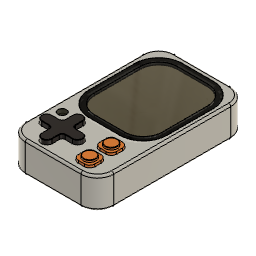
MVP Mecanico v1 (Autodesk Fusion 360 design; units mm, degrees)
Autodesk Fusion 360 part; units mm, degrees
(part 1 of 2)
sketch "Boceto1" plane through (0, 0, 0) normal (0, 0, 1) x (1, 0, 0)
  line L0 (7.34, -20.255) -> (-7.34, -20.255)
  line L1 (-16.54, -11.055) -> (-16.54, 11.055)
  line L2 (-7.34, 20.255) -> (7.34, 20.255)
  line L3 (16.54, 11.055) -> (16.54, -11.055)
  line L4 (16.54, -20.255) -> (-16.54, 20.255) construction
  line L5 (-16.54, -20.255) -> (16.54, 20.255) construction
  line L6 (8.265, -22.225) -> (-8.265, -22.225)
  line L7 (-17.465, -13.025) -> (-17.465, 11.855)
  line L8 (-8.265, 21.055) -> (8.265, 21.055)
  line L9 (17.465, 11.855) -> (17.465, -13.025)
  arc A0 (-7.34, 20.255) -> (-16.54, 11.055) centre (-7.34, 11.055) ccw
  arc A1 (16.54, 11.055) -> (7.34, 20.255) centre (7.34, 11.055) ccw
  arc A2 (-16.54, -11.055) -> (-7.34, -20.255) centre (-7.34, -11.055) ccw
  arc A3 (7.34, -20.255) -> (16.54, -11.055) centre (7.34, -11.055) ccw
  arc A4 (-8.265, 21.055) -> (-17.465, 11.855) centre (-8.265, 11.855) ccw
  arc A5 (17.465, 11.855) -> (8.265, 21.055) centre (8.265, 11.855) ccw
  arc A6 (-17.465, -13.025) -> (-8.265, -22.225) centre (-8.265, -13.025) ccw
  arc A7 (8.265, -22.225) -> (17.465, -13.025) centre (8.265, -13.025) ccw
  dimension "d3" = 33.08
  dimension "d4" = 40.51
  dimension "d7" = 9.2
  dimension "d8" = 9.2
  dimension "d9" = 9.2
  dimension "d10" = 9.2
  dimension "d11" = 9.2
  dimension "d12" = 9.2
  dimension "d13" = 9.2
  dimension "d14" = 9.2
  dimension "d15" = 0.8
  dimension "d16" = 43.28
  dimension "d17" = 34.93
  dimension "d18" = 0.925
  constraint horizontal L0
  constraint perpendicular L0 L1
  constraint parallel L0 L2
  constraint parallel L1 L3
  constraint coincident L4 origin
  constraint coincident L5 origin
  constraint horizontal L6
  constraint perpendicular L6 L7
  constraint parallel L6 L8
  constraint parallel L7 L9
  constraint coincident L4.end L1
  constraint coincident L4.end L2
  constraint tangent L1 A0
  constraint tangent L2 A0
  constraint coincident L5.end L2
  constraint coincident L5.end L3
  constraint tangent L2 A1
  constraint tangent L3 A1
  constraint coincident L5.start L1
  constraint coincident L5.start L0
  constraint tangent L1 A2
  constraint tangent L0 A2
  constraint coincident L4.start L0
  constraint coincident L4.start L3
  constraint tangent L0 A3
  constraint tangent L3 A3
  constraint tangent L7 A4
  constraint tangent L8 A4
  constraint tangent L8 A5
  constraint tangent L9 A5
  constraint tangent L7 A6
  constraint tangent L6 A6
  constraint tangent L6 A7
  constraint tangent L9 A7
  measures "d3" distance of L4.end L5.end
  measures "d4" distance of L5.start L4.end
  measures "d7" radius of A0
  measures "d8" radius of A1
  measures "d9" radius of A2
  measures "d10" radius of A3
  measures "d11" radius of A4
  measures "d12" radius of A5
  measures "d13" radius of A6
  measures "d14" radius of A7
  measures "d15" distance of L2 L8
  measures "d16" distance of L6 L8
  measures "d17" distance of L7 L9
  measures "d18" distance of L1 L7
extrude "Extruir1" add sketch "Boceto1" along normal blind 0.83 makes body 1
extrude "Extruir2" add sketch "Boceto1" along normal blind 1.03 contours L0 L1 L2 L3 A0 A1 A2 A3 bodies 1
sketch "Boceto2" plane through (0, 0, 1.03) normal (0, 0, 1) x (-1, 0, 0)
  line L0 (-7.395, 20.305) -> (7.395, 20.305)
  line L1 (16.595, 11.105) -> (16.595, -11.105)
  line L2 (7.395, -20.305) -> (-7.395, -20.305)
  line L3 (-16.595, -11.105) -> (-16.595, 11.105)
  line L4 (-16.595, 20.305) -> (16.595, -20.305) construction
  line L5 (16.595, 20.305) -> (-16.595, -20.305) construction
  arc A0 (7.395, -20.305) -> (16.595, -11.105) centre (7.395, -11.105) ccw
  arc A1 (-16.595, -11.105) -> (-7.395, -20.305) centre (-7.395, -11.105) ccw
  arc A2 (16.595, 11.105) -> (7.395, 20.305) centre (7.395, 11.105) ccw
  arc A3 (-7.395, 20.305) -> (-16.595, 11.105) centre (-7.395, 11.105) ccw
  line L6 (-7.545, 22.755) -> (7.545, 22.755)
  line L7 (19.045, 11.255) -> (19.045, -11.255)
  line L8 (7.545, -22.755) -> (-7.545, -22.755)
  line L9 (-19.045, -11.255) -> (-19.045, 11.255)
  line L10 (-19.045, 22.755) -> (19.045, -22.755) construction
  line L11 (19.045, 22.755) -> (-19.045, -22.755) construction
  arc A4 (7.545, -22.755) -> (19.045, -11.255) centre (7.545, -11.255) ccw
  arc A5 (-19.045, -11.255) -> (-7.545, -22.755) centre (-7.545, -11.255) ccw
  arc A6 (19.045, 11.255) -> (7.545, 22.755) centre (7.545, 11.255) ccw
  arc A7 (-7.545, 22.755) -> (-19.045, 11.255) centre (-7.545, 11.255) ccw
  dimension "d30" = 40.61
  dimension "d31" = 33.19
  dimension "d32" = 9.2
  dimension "d33" = 9.2
  dimension "d34" = 9.2
  dimension "d35" = 9.2
  dimension "d36" = 45.51
  dimension "d37" = 38.09
  dimension "d38" = 11.5
  dimension "d39" = 11.5
  dimension "d40" = 11.5
  dimension "d41" = 11.5
  constraint horizontal L0
  constraint perpendicular L0 L1
  constraint parallel L0 L2
  constraint parallel L1 L3
  constraint coincident L4 origin
  constraint coincident L5 origin
  constraint coincident L4.end L1
  constraint coincident L4.end L2
  constraint tangent L1 A0
  constraint tangent L2 A0
  constraint coincident L5.end L2
  constraint coincident L5.end L3
  constraint tangent L2 A1
  constraint tangent L3 A1
  constraint coincident L5.start L1
  constraint coincident L5.start L0
  constraint tangent L1 A2
  constraint tangent L0 A2
  constraint coincident L4.start L0
  constraint coincident L4.start L3
  constraint tangent L0 A3
  constraint tangent L3 A3
  constraint horizontal L6
  constraint perpendicular L6 L7
  constraint parallel L6 L8
  constraint parallel L7 L9
  constraint coincident L10 origin
  constraint coincident L11 origin
  constraint coincident L10.end L7
  constraint coincident L10.end L8
  constraint tangent L7 A4
  constraint tangent L8 A4
  constraint coincident L11.end L8
  constraint coincident L11.end L9
  constraint tangent L8 A5
  constraint tangent L9 A5
  constraint coincident L11.start L7
  constraint coincident L11.start L6
  constraint tangent L7 A6
  constraint tangent L6 A6
  constraint coincident L10.start L6
  constraint coincident L10.start L9
  constraint tangent L6 A7
  constraint tangent L9 A7
  measures "d30" distance of L5.start L4.end
  measures "d31" distance of L4.end L5.end
  measures "d32" radius of A0
  measures "d33" radius of A1
  measures "d34" radius of A2
  measures "d35" radius of A3
  measures "d36" distance of L11.start L10.end
  measures "d37" distance of L10.end L11.end
  measures "d38" radius of A4
  measures "d39" radius of A5
  measures "d40" radius of A6
  measures "d41" radius of A7
sketch "Boceto3" plane through (0, 0, 0.83) normal (0, 0, 1) x (-1, 0, 0)
  arc A0 (17.465, 13.025) -> (8.265, 22.225) centre (8.265, 13.025) ccw
  line L0 (8.265, 22.225) -> (-8.265, 22.225)
  arc A1 (-8.265, 22.225) -> (-17.465, 13.025) centre (-8.265, 13.025) ccw
  line L1 (-17.465, 13.025) -> (-17.465, -11.855)
  arc A2 (-17.465, -11.855) -> (-8.265, -21.055) centre (-8.265, -11.855) ccw
  line L2 (-8.265, -21.055) -> (8.265, -21.055)
  arc A3 (8.265, -21.055) -> (17.465, -11.855) centre (8.265, -11.855) ccw
  line L3 (17.465, -11.855) -> (17.465, 13.025)
  line L4 (11.3983, 21.675) -> (-11.3983, 21.675)
  arc A4 (16.54, 11.055) -> (7.34, 20.255) centre (7.34, 11.055) ccw
  line L5 (16.54, 11.055) -> (16.54, -11.055)
  arc A5 (7.34, -20.255) -> (16.54, -11.055) centre (7.34, -11.055) ccw
  line L6 (7.34, -20.255) -> (-7.34, -20.255)
  arc A6 (-16.54, -11.055) -> (-7.34, -20.255) centre (-7.34, -11.055) ccw
  line L7 (-16.54, -11.055) -> (-16.54, 11.055)
  arc A7 (-7.34, 20.255) -> (-16.54, 11.055) centre (-7.34, 11.055) ccw
  line L8 (-7.34, 20.255) -> (7.34, 20.255)
  dimension "d42" = 0.55
  constraint coincident A0 L4.start
  constraint coincident A1 L4.end
  constraint horizontal L4
  measures "d42" distance of L0 L4
extrude "Extruir3" cut sketch "Boceto3" against normal blind 0.4 contours A0 L0 A1 L4 bodies 1
extrude "Extruir4" add sketch "Boceto2" along normal blind 1.1 separate body makes body 2
extrude "Extruir5" add 1 faces at (-5.5133, -3.685, 1.03) along direction (0, 0, 1) blind 1.1 separate body on bodies 1 makes body 3
sketch "Boceto4" plane through (0, 0, 1.03) normal (0, 0, -1) x (1, 0, 0)
  arc A0 (-7.395, 20.305) -> (-16.595, 11.105) centre (-7.395, 11.105) ccw
  line L0 (-7.395, 20.305) -> (7.395, 20.305)
  arc A1 (16.595, 11.105) -> (7.395, 20.305) centre (7.395, 11.105) ccw
  line L1 (16.595, 11.105) -> (16.595, -11.105)
  arc A2 (7.395, -20.305) -> (16.595, -11.105) centre (7.395, -11.105) ccw
  line L2 (7.395, -20.305) -> (-7.395, -20.305)
  arc A3 (-16.595, -11.105) -> (-7.395, -20.305) centre (-7.395, -11.105) ccw
  line L3 (-16.595, -11.105) -> (-16.595, 11.105)
  arc A4 (-7.545, 22.755) -> (-19.045, 11.255) centre (-7.545, 11.255) ccw
  line L4 (-19.045, 11.255) -> (-19.045, -11.255)
  arc A5 (-19.045, -11.255) -> (-7.545, -22.755) centre (-7.545, -11.255) ccw
  line L5 (-7.545, -22.755) -> (7.545, -22.755)
  arc A6 (7.545, -22.755) -> (19.045, -11.255) centre (7.545, -11.255) ccw
  line L6 (19.045, -11.255) -> (19.045, 11.255)
  arc A7 (19.045, 11.255) -> (7.545, 22.755) centre (7.545, 11.255) ccw
  line L7 (7.545, 22.755) -> (-7.545, 22.755)
  line L8 (-8.265, 22.425) -> (8.265, 22.425)
  line L9 (17.665, 13.025) -> (17.665, -11.855)
  line L10 (8.265, -21.255) -> (-8.265, -21.255)
  line L11 (-17.665, -11.855) -> (-17.665, 13.025)
  line L12 (8.265, 22.225) -> (-8.265, 22.225)
  arc A8 (8.265, -21.255) -> (17.665, -11.855) centre (8.265, -11.855) ccw
  arc A9 (-17.665, -11.855) -> (-8.265, -21.255) centre (-8.265, -11.855) ccw
  arc A10 (17.665, 13.025) -> (8.265, 22.425) centre (8.265, 13.025) ccw
  arc A11 (-8.265, 22.425) -> (-17.665, 13.025) centre (-8.265, 13.025) ccw
  line L13 (-8.45, 25) -> (8.45, 25)
  line L14 (20, 13.45) -> (20, -13.45)
  line L15 (8.45, -25) -> (-8.45, -25)
  line L16 (-20, -13.45) -> (-20, 13.45)
  line L17 (-20, 25) -> (20, -25) construction
  line L18 (20, 25) -> (-20, -25) construction
  arc A12 (20, 13.45) -> (8.45, 25) centre (8.45, 13.45) ccw
  arc A13 (-8.45, 25) -> (-20, 13.45) centre (-8.45, 13.45) ccw
  arc A14 (8.45, -25) -> (20, -13.45) centre (8.45, -13.45) ccw
  arc A15 (-20, -13.45) -> (-8.45, -25) centre (-8.45, -13.45) ccw
  dimension "d52" = 0.2
  dimension "d55" = 9.4
  dimension "d56" = 9.4
  dimension "d57" = 9.4
  dimension "d58" = 9.4
  dimension "d59" = 40
  dimension "d60" = 50
  dimension "d61" = 11.55
  dimension "d62" = 11.55
  dimension "d63" = 11.55
  dimension "d64" = 11.55
  constraint horizontal L8
  constraint perpendicular L8 L9
  constraint parallel L8 L10
  constraint parallel L9 L11
  constraint tangent L9 A8
  constraint tangent L10 A8
  constraint tangent L10 A9
  constraint tangent L11 A9
  constraint tangent L9 A10
  constraint tangent L8 A10
  constraint tangent L8 A11
  constraint tangent L11 A11
  constraint horizontal L13
  constraint perpendicular L13 L14
  constraint parallel L13 L15
  constraint parallel L14 L16
  constraint coincident L17 origin
  constraint coincident L18 origin
  constraint coincident L18.start L14
  constraint coincident L18.start L13
  constraint tangent L14 A12
  constraint tangent L13 A12
  constraint coincident L17.start L13
  constraint coincident L17.start L16
  constraint tangent L13 A13
  constraint tangent L16 A13
  constraint coincident L17.end L15
  constraint coincident L17.end L14
  constraint tangent L15 A14
  constraint tangent L14 A14
  constraint coincident L18.end L15
  constraint coincident L18.end L16
  constraint tangent L15 A15
  constraint tangent L16 A15
  measures "d52" distance of L8 L12
  measures "d55" radius of A8
  measures "d56" radius of A9
  measures "d57" radius of A10
  measures "d58" radius of A11
  measures "d59" distance of L17.end L18.end
  measures "d60" distance of L18.start L17.end
  measures "d61" radius of A12
  measures "d62" radius of A13
  measures "d63" radius of A14
  measures "d64" radius of A15
sketch "Boceto5" plane through (0, 0, 2.13) normal (0, 0, 1) x (-1, 0, 0)
  arc A0 (16.595, 11.105) -> (7.395, 20.305) centre (7.395, 11.105) ccw
  line L0 (16.595, 11.105) -> (16.595, -11.105)
  arc A1 (7.395, -20.305) -> (16.595, -11.105) centre (7.395, -11.105) ccw
  line L1 (7.395, -20.305) -> (-7.395, -20.305)
  arc A2 (-16.595, -11.105) -> (-7.395, -20.305) centre (-7.395, -11.105) ccw
  line L2 (-16.595, -11.105) -> (-16.595, 11.105)
  arc A3 (-7.395, 20.305) -> (-16.595, 11.105) centre (-7.395, 11.105) ccw
  line L3 (-7.395, 20.305) -> (7.395, 20.305)
  arc A4 (19.045, 11.255) -> (7.545, 22.755) centre (7.545, 11.255) ccw
  line L4 (7.545, 22.755) -> (-7.545, 22.755)
  arc A5 (-7.545, 22.755) -> (-19.045, 11.255) centre (-7.545, 11.255) ccw
  line L5 (-19.045, 11.255) -> (-19.045, -11.255)
  arc A6 (-19.045, -11.255) -> (-7.545, -22.755) centre (-7.545, -11.255) ccw
  line L6 (-7.545, -22.755) -> (7.545, -22.755)
  arc A7 (7.545, -22.755) -> (19.045, -11.255) centre (7.545, -11.255) ccw
  line L7 (19.045, -11.255) -> (19.045, 11.255)
  line L8 (-7.57, 22.83) -> (7.57, 22.83)
  line L9 (19.12, 11.28) -> (19.12, -11.28)
  line L10 (7.57, -22.83) -> (-7.57, -22.83)
  line L11 (-19.12, -11.28) -> (-19.12, 11.28)
  line L12 (-19.12, 22.83) -> (19.12, -22.83) construction
  line L13 (19.12, 22.83) -> (-19.12, -22.83) construction
  arc A8 (7.57, -22.83) -> (19.12, -11.28) centre (7.57, -11.28) ccw
  arc A9 (-19.12, -11.28) -> (-7.57, -22.83) centre (-7.57, -11.28) ccw
  arc A10 (19.12, 11.28) -> (7.57, 22.83) centre (7.57, 11.28) ccw
  arc A11 (-7.57, 22.83) -> (-19.12, 11.28) centre (-7.57, 11.28) ccw
  line L14 (-13.52, -25.28) -> (13.57, -25.28)
  line L15 (21.57, -17.28) -> (21.57, 39.73)
  line L16 (13.57, 47.73) -> (-13.52, 47.73)
  line L17 (-21.52, 39.73) -> (-21.52, -17.28)
  line L18 (-21.52, -25.28) -> (21.57, 47.73) construction
  line L19 (21.57, -25.28) -> (-21.52, 47.73) construction
  arc A12 (13.57, -25.28) -> (21.57, -17.28) centre (13.57, -17.28) ccw
  arc A13 (-21.52, -17.28) -> (-13.52, -25.28) centre (-13.52, -17.28) ccw
  arc A14 (21.57, 39.73) -> (13.57, 47.73) centre (13.57, 39.73) ccw
  arc A15 (-13.52, 47.73) -> (-21.52, 39.73) centre (-13.52, 39.73) ccw
  point P0 (0.025, 11.225)
  dimension "d67" = 45.66
  dimension "d68" = 38.24
  dimension "d69" = 11.55
  dimension "d70" = 11.55
  dimension "d71" = 11.55
  dimension "d72" = 11.55
  dimension "d76" = 73.01
  dimension "d77" = 8
  dimension "d78" = 8
  dimension "d79" = 8
  dimension "d80" = 8
  dimension "d234" = 43.09
  constraint horizontal L8
  constraint perpendicular L8 L9
  constraint parallel L8 L10
  constraint parallel L9 L11
  constraint coincident L12 origin
  constraint coincident L13 origin
  constraint coincident L12.end L9
  constraint coincident L12.end L10
  constraint tangent L9 A8
  constraint tangent L10 A8
  constraint coincident L13.end L10
  constraint coincident L13.end L11
  constraint tangent L10 A9
  constraint tangent L11 A9
  constraint coincident L13.start L9
  constraint coincident L13.start L8
  constraint tangent L9 A10
  constraint tangent L8 A10
  constraint coincident L12.start L8
  constraint coincident L12.start L11
  constraint tangent L8 A11
  constraint tangent L11 A11
  constraint horizontal L14
  constraint perpendicular L14 L15
  constraint parallel L14 L16
  constraint parallel L15 L17
  constraint coincident L18 P0
  constraint coincident L19 P0
  constraint coincident L19.start L15
  constraint coincident L19.start L14
  constraint tangent L15 A12
  constraint tangent L14 A12
  constraint coincident L18.start L14
  constraint coincident L18.start L17
  constraint tangent L14 A13
  constraint tangent L17 A13
  constraint coincident L18.end L15
  constraint coincident L18.end L16
  constraint tangent L15 A14
  constraint tangent L16 A14
  constraint coincident L19.end L17
  constraint coincident L19.end L16
  constraint tangent L17 A15
  constraint tangent L16 A15
  measures "d67" distance of L13.start L12.end
  measures "d68" distance of L12.end L13.end
  measures "d69" radius of A8
  measures "d70" radius of A9
  measures "d71" radius of A10
  measures "d72" radius of A11
  measures "d76" distance of L19.start L18.end
  measures "d77" radius of A12
  measures "d78" radius of A13
  measures "d79" radius of A14
  measures "d80" radius of A15
  measures "d234" distance of L15 L17
extrude "Extruir7" add sketch "Boceto5" against normal blind 2 separate body contours L14 L15 L16 L17 A12 A13 A14 A15 makes body 4
sketch "Boceto6" plane through (0, 0, 0.13) normal (0, 0, -1) x (1, 0, 0)
  arc A0 (-7.57, 22.83) -> (-19.12, 11.28) centre (-7.57, 11.28) ccw
  line L0 (-7.57, 22.83) -> (7.57, 22.83)
  arc A1 (19.12, 11.28) -> (7.57, 22.83) centre (7.57, 11.28) ccw
  line L1 (19.12, 11.28) -> (19.12, -11.28)
  arc A2 (7.57, -22.83) -> (19.12, -11.28) centre (7.57, -11.28) ccw
  line L2 (7.57, -22.83) -> (-7.57, -22.83)
  arc A3 (-19.12, -11.28) -> (-7.57, -22.83) centre (-7.57, -11.28) ccw
  line L3 (-19.12, -11.28) -> (-19.12, 11.28)
  arc A4 (21.52, 39.73) -> (13.52, 47.73) centre (13.52, 39.73) ccw
  line L4 (13.52, 47.73) -> (-13.57, 47.73)
  arc A5 (-13.57, 47.73) -> (-21.57, 39.73) centre (-13.57, 39.73) ccw
  line L5 (-21.57, 39.73) -> (-21.57, -17.28)
  arc A6 (-21.57, -17.28) -> (-13.57, -25.28) centre (-13.57, -17.28) ccw
  line L6 (-13.57, -25.28) -> (13.52, -25.28)
  arc A7 (13.52, -25.28) -> (21.52, -17.28) centre (13.52, -17.28) ccw
  line L7 (21.52, -17.28) -> (21.52, 39.73)
  line L8 (-13.57, -23.78) -> (13.52, -23.78)
  arc A8 (13.52, -23.78) -> (20.02, -17.28) centre (13.52, -17.28) ccw
  line L9 (20.02, -17.28) -> (20.02, 39.73)
  arc A9 (20.02, 39.73) -> (13.52, 46.23) centre (13.52, 39.73) ccw
  line L10 (13.52, 46.23) -> (-13.57, 46.23)
  arc A10 (-13.57, 46.23) -> (-20.07, 39.73) centre (-13.57, 39.73) ccw
  line L11 (-20.07, 39.73) -> (-20.07, -17.28)
  arc A11 (-20.07, -17.28) -> (-13.57, -23.78) centre (-13.57, -17.28) ccw
  dimension "d83" = -1.5
extrude "Extruir8" add sketch "Boceto6" along normal blind 13 contours A4 L4 A5 L5 A6 L6 A7 L7 bodies 4
fillet "Empalme1" radius 1 8 edges at (21.52, -11.225, 2.13) (19.1769, 22.9369, 2.13) (-0.025, 25.28, 2.13) (-19.2269, 22.9369, 2.13) (-21.57, -11.225, 2.13) (-19.2269, -45.3869, 2.13) (-0.025, -47.73, 2.13) (19.1769, -45.3869, 2.13) on bodies 4
fillet "Empalme2" radius 1 8 edges at (-21.57, -11.225, -12.87) (-19.2269, 22.9369, -12.87) (-0.025, 25.28, -12.87) (19.1769, 22.9369, -12.87) (21.52, -11.225, -12.87) (19.1769, -45.3869, -12.87) (-0.025, -47.73, -12.87) (-19.2269, -45.3869, -12.87) on bodies 4
extrude "Extruir9" add sketch "Boceto4" along normal up to surface (0.9 mm away) separate body contours A4 L4 A5 L5 A6 L6 A7 L7 | L13 L14 L15 L16 A12 A13 A14 A15 makes body 5
ref_plane "PlanoDeObra1" through (-0.025, -11.225, -10.34) normal (0, 0, -1) x (1, 0, 0)
sketch "Boceto7" plane through (0, 0, -10.34) normal (0, 0, -1) x (-1, 0, 0)
  line L0 (-13.52, -47.73) -> (13.57, -47.73)
  line L1 (-21.52, 17.28) -> (-21.52, -39.73)
  circle A0 centre (-15.52, -41.73) radius 1.4
  line L2 (20.07, -11.225) -> (-20.02, -11.225) construction
  line L3 (-20.02, -39.73) -> (-20.02, 17.28)
  line L4 (20.07, 17.28) -> (20.07, -39.73)
  line L5 (0.025, -46.23) -> (0.025, 23.78) construction
  line L6 (13.57, -46.23) -> (-13.52, -46.23)
  line L7 (-13.52, 23.78) -> (13.57, 23.78)
  line L8 (-13.52, -46.23) -> (-20.02, -46.23) construction
  line L9 (-20.02, -39.73) -> (-20.02, -46.23) construction
  line L10 (-20.02, -46.23) -> (-16.036, -42.6017) construction
  line L11 (-13.5, -43.948) -> (-17.54, -39.512) construction
  arc A1 (-13.5, -43.948) -> (-17.54, -39.512) centre (-15.52, -41.73) ccw
  arc A2 (-20.02, -39.73) -> (-13.52, -46.23) centre (-14.0388, -40.2488) ccw
  line L12 (-13.5, -43.948) -> (-15.7552, -46.0019)
  line L13 (-17.54, -39.512) -> (-19.8786, -41.6418)
  circle A3 centre (-15.52, 19.28) radius 1.4
  line L14 (-13.5, 21.498) -> (-15.7552, 23.5519)
  arc A4 (-17.54, 17.062) -> (-13.5, 21.498) centre (-15.52, 19.28) ccw
  line L15 (-17.54, 17.062) -> (-19.8786, 19.1918)
  arc A5 (-13.52, 23.78) -> (-20.02, 17.28) centre (-14.0388, 17.7988) ccw
  circle A6 centre (15.57, 19.28) radius 1.4
  line L16 (17.59, 17.062) -> (19.9286, 19.1918)
  arc A7 (13.55, 21.498) -> (17.59, 17.062) centre (15.57, 19.28) ccw
  line L17 (13.55, 21.498) -> (15.8052, 23.5519)
  arc A8 (20.07, 17.28) -> (13.57, 23.78) centre (14.0888, 17.7988) ccw
  line L18 (13.55, -43.948) -> (15.8052, -46.0019)
  arc A9 (17.59, -39.512) -> (13.55, -43.948) centre (15.57, -41.73) ccw
  circle A10 centre (15.57, -41.73) radius 1.4
  line L19 (17.59, -39.512) -> (19.9286, -41.6418)
  arc A11 (13.57, -46.23) -> (20.07, -39.73) centre (14.0888, -40.2488) ccw
  dimension "d93" = 6
  dimension "d94" = 6
  dimension "d96" = 2.8
  dimension "d97" = 6
  constraint horizontal L2
  constraint midpoint L2.end L3
  constraint coincident L2.start L4
  constraint vertical L5
  constraint midpoint L5.start L6
  constraint midpoint L5.end L7
  constraint concentric A0 A1
  constraint coincident L6.end L8.start
  constraint parallel L6 L8
  constraint coincident L3.start L9.start
  constraint perpendicular L8 L9
  constraint perpendicular L10 L11
  constraint midpoint A0.centre L11
  constraint coincident A2 L12.end
  constraint tangent A1 L12
  constraint coincident A2 L13.end
  constraint tangent A1 L13
  constraint symmetric A0 L2 A3
  constraint symmetric L2 L11.start L14.start
  constraint symmetric L2 L11.end A4.start
  constraint symmetric L2 A1 A4
  constraint symmetric L2 L6.end L7.start
  constraint symmetric L2 L3.start L3.end
  constraint symmetric L2 A2 A5
  constraint symmetric L2 L12.end L14.end
  constraint symmetric L2 L13.end L15.end
  constraint symmetric A0 L5 A10
  constraint symmetric L5 L11.start L18.start
  constraint symmetric L5 L11.end A9.start
  constraint symmetric L5 A1 A9
  constraint symmetric L5 L6.end L6.start
  constraint symmetric L5 L3.start L4.end
  constraint symmetric L5 A2 A11
  constraint symmetric L5 L12.end L18.end
  constraint symmetric L5 L13.end L19.end
  constraint symmetric L5 A3 A6
  constraint symmetric L5 L14.start A7.start
  constraint symmetric L5 L14.end L17.end
  constraint symmetric L5 A4.start L16.start
  constraint symmetric L5 A4 A7
  constraint symmetric L5 L15.end L16.end
  constraint symmetric L5 L3.end L4.start
  constraint symmetric L5 L7.start L7.end
  constraint symmetric L5 A5 A8
  measures "d93" distance of L0 A0.centre
  measures "d94" distance of L1 A0.centre
  measures "d96" diameter of A0
  measures "d97" diameter of A1
extrude "Extruir10" add sketch "Boceto7" against normal blind 3 separate body contours A1 A2 L12 L13 | L14 A4 L15 A5 | L18 A9 L19 A11 | L16 A7 L17 A8 makes body 6 at (18.0921, -40.8237, -10.34) makes body 7 at (-18.1421, 18.3737, -10.34) makes body 8 at (-18.1421, -40.8237, -10.34) makes body 9 at (18.0921, 18.3737, -10.34)
sketch "Boceto8" plane through (0, 0, -12.87) normal (0, 0, -1) x (1, 0, 0)
  arc A0 (-20.07, -17.28) -> (-13.57, -23.78) centre (-13.57, -17.28) ccw
  line L0 (-20.07, -17.28) -> (-20.07, 39.73)
  arc A1 (-13.57, 46.23) -> (-20.07, 39.73) centre (-13.57, 39.73) ccw
  line L1 (-13.57, 46.23) -> (13.52, 46.23)
  arc A2 (20.02, 39.73) -> (13.52, 46.23) centre (13.52, 39.73) ccw
  line L2 (20.02, 39.73) -> (20.02, -17.28)
  arc A3 (13.52, -23.78) -> (20.02, -17.28) centre (13.52, -17.28) ccw
  line L3 (13.52, -23.78) -> (-13.57, -23.78)
  line L4 (-20.57, 39.73) -> (-20.57, -17.28)
  arc A4 (-20.57, -17.28) -> (-13.57, -24.28) centre (-13.57, -17.28) ccw
  line L5 (-13.57, -24.28) -> (13.52, -24.28)
  arc A5 (13.52, -24.28) -> (20.52, -17.28) centre (13.52, -17.28) ccw
  line L6 (20.52, -17.28) -> (20.52, 39.73)
  arc A6 (20.52, 39.73) -> (13.52, 46.73) centre (13.52, 39.73) ccw
  line L7 (13.52, 46.73) -> (-13.57, 46.73)
  arc A7 (-13.57, 46.73) -> (-20.57, 39.73) centre (-13.57, 39.73) ccw
  line L8 (-19.97, -17.28) -> (-19.97, 39.73)
  arc A8 (-13.57, 46.13) -> (-19.97, 39.73) centre (-13.57, 39.73) ccw
  line L9 (-13.57, 46.13) -> (13.52, 46.13)
  arc A9 (19.92, 39.73) -> (13.52, 46.13) centre (13.52, 39.73) ccw
  line L10 (19.92, 39.73) -> (19.92, -17.28)
  arc A10 (13.52, -23.68) -> (19.92, -17.28) centre (13.52, -17.28) ccw
  line L11 (13.52, -23.68) -> (-13.57, -23.68)
  arc A11 (-19.97, -17.28) -> (-13.57, -23.68) centre (-13.57, -17.28) ccw
  circle A12 centre (-15.57, -19.28) radius 1.3
  line L12 (-13.57, -25.28) -> (13.52, -25.28)
  line L13 (-21.57, 39.73) -> (-21.57, -17.28)
  circle A13 centre (-15.57, -19.28) radius 2.15
  line L14 (19.92, 11.225) -> (-19.97, 11.225) construction
  line L15 (-0.025, -23.68) -> (-0.025, 46.13) construction
  line L16 (-0.025, 46.13) -> (-0.025, -23.68) construction
  line L17 (19.92, 11.225) -> (-19.97, 11.225) construction
  circle A14 centre (-15.57, 41.73) radius 2.15
  circle A15 centre (-15.57, 41.73) radius 1.3
  circle A16 centre (15.52, -19.28) radius 1.3
  circle A17 centre (15.52, -19.28) radius 2.15
  circle A18 centre (15.52, 41.73) radius 2.15
  circle A19 centre (15.52, 41.73) radius 1.3
  dimension "d100" = 0.1
  dimension "d101" = 2.6
  dimension "d104" = 6
  dimension "d105" = 6
  dimension "d106" = 4.3
  constraint concentric A12 A13
  constraint horizontal L14
  constraint midpoint L8 L14.end
  constraint midpoint L10 L14.start
  constraint vertical L15
  constraint midpoint L11 L15.start
  constraint midpoint L9 L15.end
  constraint symmetric A12 L14 A15
  constraint symmetric A13 L14 A14
  constraint symmetric L17.start L14 L14.start
  constraint symmetric L17.end L14 L14.end
  constraint symmetric L14 L15.start L15.end
  constraint symmetric L14 L15.end L15.start
  constraint symmetric A12 L15 A16
  constraint symmetric A13 L15 A17
  constraint symmetric L15 A14 A18
  constraint symmetric L15 A15 A19
  measures "d101" diameter of A12
  measures "d104" distance of A12.centre L12
  measures "d105" distance of A12.centre L13
  measures "d106" diameter of A13
extrude "Extruir11" add sketch "Boceto8" against normal blind 2.52 separate body contours L8 A8 L9 A9 L10 A10 L11 A11 | A13 | A14 | A17 | A18 makes body 10
extrude "Extruir12" cut sketch "Boceto8" against normal blind 1.73 contours A13 | A14 | A17 | A18 bodies 10
ref_plane "PlanoDeObra2" through (-0.025, -11.225, -4.87) normal (0, 0, -1) x (1, 0, 0)
sketch "Boceto9" plane through (0, 0, -4.87) normal (0, 0, -1) x (-1, 0, 0)
  line L0 (5.025, 21.78) -> (-4.975, 21.78)
  line L1 (-4.975, 21.78) -> (-4.975, 23.78)
  line L2 (-4.975, 23.78) -> (5.025, 23.78)
  line L3 (5.025, 23.78) -> (5.025, 21.78)
  line L4 (5.025, 21.78) -> (-4.975, 23.78) construction
  line L5 (-4.975, 21.78) -> (5.025, 23.78) construction
  line L6 (-13.52, 23.78) -> (13.57, 23.78)
  line L7 (-20.02, -11.225) -> (20.07, -11.225) construction
  line L8 (20.07, 17.28) -> (20.07, -39.73)
  line L9 (-20.02, -39.73) -> (-20.02, 17.28)
  line L10 (0.025, 23.78) -> (0.025, -46.23) construction
  line L11 (13.57, -46.23) -> (-13.52, -46.23)
  line L12 (-4.975, -44.23) -> (-4.975, -46.23)
  line L13 (-4.975, -46.23) -> (5.025, -46.23)
  line L14 (5.025, -44.23) -> (-4.975, -44.23)
  line L15 (5.025, -46.23) -> (5.025, -44.23)
  line L16 (20.07, -16.225) -> (18.07, -16.225)
  line L17 (18.07, -16.225) -> (18.07, -6.225)
  line L18 (18.07, -6.225) -> (20.07, -6.225)
  line L19 (20.07, -6.225) -> (20.07, -16.225)
  line L20 (20.07, -16.225) -> (18.07, -6.225) construction
  line L21 (18.07, -16.225) -> (20.07, -6.225) construction
  line L22 (-20.02, -16.225) -> (-18.02, -16.225)
  line L23 (-18.02, -16.225) -> (-18.02, -6.225)
  line L24 (-18.02, -6.225) -> (-20.02, -6.225)
  line L25 (-20.02, -6.225) -> (-20.02, -16.225)
  point P0 (0.025, 22.78)
  point P1 (19.07, -11.225)
  dimension "d112" = 2
  dimension "d113" = 10
  dimension "d114" = 2
  dimension "d115" = 10
  constraint horizontal L0
  constraint perpendicular L0 L1
  constraint parallel L0 L2
  constraint parallel L1 L3
  constraint coincident L4 P0
  constraint coincident L5 P0
  constraint midpoint L2 L6
  constraint horizontal L7
  constraint midpoint L7.end L8
  constraint midpoint L7.start L9
  constraint perpendicular L7 L10
  constraint midpoint L2 L10.start
  constraint midpoint L10.end L11
  constraint symmetric L0.start L7 L14.start
  constraint symmetric L0.end L7 L12.start
  constraint symmetric L1.end L7 L12.end
  constraint symmetric L2.end L7 L13.end
  constraint horizontal L16
  constraint perpendicular L16 L17
  constraint parallel L16 L18
  constraint parallel L17 L19
  constraint coincident L20 P1
  constraint coincident L21 P1
  constraint midpoint L8 L19
  constraint symmetric L10 L16.start L22.start
  constraint symmetric L10 L16.end L22.end
  constraint symmetric L10 L17.end L23.end
  constraint symmetric L10 L18.end L24.end
  measures "d112" distance of L0.end L1.end
  measures "d113" distance of L0.start L0.end
  measures "d114" distance of L17.end L18.end
  measures "d115" distance of L16.end L17.end
extrude "Extruir13" add sketch "Boceto9" against normal blind 2 bodies 7 8 6 9 4
sketch "Boceto10" plane through (0, 0, -4.87) normal (0, 0, -1) x (1, 0, 0)
  line L0 (-5.025, 46.23) -> (-5.025, 44.23)
  line L1 (-5.025, 44.23) -> (4.975, 44.23)
  line L2 (4.975, 44.23) -> (4.975, 46.23)
  line L3 (4.975, 46.23) -> (-5.025, 46.23)
  line L4 (20.02, 11.225) -> (-20.07, 11.225) construction
  line L5 (20.02, 39.73) -> (20.02, -17.28)
  line L6 (-20.07, -17.28) -> (-20.07, 39.73)
  line L7 (-0.025, 46.23) -> (-0.025, -23.78) construction
  line L8 (13.52, -23.78) -> (-13.57, -23.78)
  arc A0 (13.5, 43.948) -> (17.54, 39.512) centre (15.52, 41.73) ccw
  line L9 (13.52, 47.73) -> (21.52, 47.73) construction
  line L10 (21.52, 47.73) -> (21.52, 39.73) construction
  line L11 (15.52, 41.73) -> (21.52, 47.73) construction
  line L12 (15.52, 41.73) -> (17.9949, 39.2551) construction
  line L13 (15.52, 41.73) -> (13.0451, 44.2049) construction
  line L14 (13.0451, 44.2049) -> (14.1874, 45.3472)
  line L15 (17.9949, 39.2551) -> (19.1372, 40.3974)
  line L16 (13.52, 47.73) -> (13.52, 46.23) construction
  line L17 (21.52, 39.73) -> (20.02, 39.73) construction
  arc A1 (14.8645, 46.0242) -> (13.52, 46.23) centre (13.2207, 39.7786) ccw
  arc A2 (13.0451, 44.2049) -> (17.9949, 39.2551) centre (15.52, 41.73) ccw
  arc A3 (20.02, 39.73) -> (13.52, 46.23) centre (13.52, 39.73) ccw
  line L18 (13.52, 46.23) -> (-0.025, 46.23)
  line L19 (-13.57, 46.23) -> (13.52, 46.23)
  line L20 (20.02, 39.73) -> (20.02, 11.225)
  line L21 (-0.025, 46.03) -> (13.9046, 46.03)
  line L22 (19.82, 11.225) -> (19.82, 40.1146)
  arc A4 (17.9949, -16.8051) -> (13.0451, -21.7549) centre (15.52, -19.28) ccw
  line L23 (17.9949, -16.8051) -> (19.15, -17.9608)
  line L24 (19.82, 11.225) -> (19.8329, -17.6778)
  line L25 (-0.025, -23.58) -> (13.9212, -23.5977)
  line L26 (13.0451, -21.7549) -> (14.2046, -22.915)
  line L27 (-0.025, -23.58) -> (-13.9546, -23.58)
  line L28 (-13.0951, -21.7549) -> (-14.2374, -22.8972)
  arc A5 (-13.0951, -21.7549) -> (-18.0449, -16.8051) centre (-15.57, -19.28) ccw
  line L29 (-18.0449, -16.8051) -> (-19.1872, -17.9474)
  line L30 (-19.87, 11.225) -> (-19.87, -17.6646)
  line L31 (-0.025, 46.03) -> (-13.9546, 46.03)
  arc A6 (-18.0449, 39.2551) -> (-13.0951, 44.2049) centre (-15.57, 41.73) ccw
  line L32 (-13.0951, 44.2049) -> (-14.2374, 45.3472)
  line L33 (-18.0449, 39.2551) -> (-19.1872, 40.3974)
  line L34 (-19.87, 11.225) -> (-19.87, 40.1146)
  arc A7 (19.82, 40.1146) -> (19.1372, 40.3974) centre (19.42, 40.1146) ccw
  arc A8 (14.1874, 45.3472) -> (13.9046, 46.03) centre (13.9046, 45.63) ccw
  arc A9 (-19.1872, 40.3974) -> (-19.87, 40.1146) centre (-19.47, 40.1146) ccw
  arc A10 (-13.9546, 46.03) -> (-14.2374, 45.3472) centre (-13.9546, 45.63) ccw
  arc A11 (-19.87, -17.6646) -> (-19.1872, -17.9474) centre (-19.47, -17.6646) ccw
  arc A12 (-14.2374, -22.8972) -> (-13.9546, -23.58) centre (-13.9546, -23.18) ccw
  arc A13 (13.9212, -23.5977) -> (14.2046, -22.915) centre (13.9217, -23.1977) ccw
  arc A14 (19.15, -17.9608) -> (19.8329, -17.6778) centre (19.4329, -17.678) ccw
  point P0 (21.52, 39.73)
  point P1 (13.52, 47.73)
  point P2 (13.52, 46.23)
  dimension "d118" = 7
  dimension "d119" = 0.2
  dimension "d120" = 0.2
  dimension "d121" = 0.4
  dimension "d122" = 0.4
  dimension "d123" = 0.4
  dimension "d124" = 0.4
  dimension "d125" = 0.4
  dimension "d126" = 0.4
  dimension "d127" = 0.4
  dimension "d128" = 0.4
  constraint horizontal L4
  constraint midpoint L4.start L5
  constraint midpoint L4.end L6
  constraint vertical L7
  constraint midpoint L3 L7.start
  constraint midpoint L7.end L8
  constraint concentric A0 A2
  constraint horizontal L9
  constraint perpendicular L9 L10
  constraint coincident P0 L10.end
  constraint coincident P1 L9.start
  constraint coincident A0.centre L11.start
  constraint perpendicular L11 L12
  constraint perpendicular L11 L13
  constraint tangent L14 A2
  constraint tangent L15 A2
  constraint perpendicular L9 L16
  constraint coincident P2 L16.end
  constraint perpendicular L10 L17
  constraint coincident L5 L17.end
  constraint tangent A3 L18
  constraint midpoint L7.start L19
  constraint coincident L5.start L17.end
  constraint coincident L5 L4.start
  constraint perpendicular L17 L20
  constraint midpoint L5 L4.start
  constraint parallel L18 L21
  constraint coincident L7 L21.start
  constraint vertical L22
  constraint coincident L4 L22.start
  constraint symmetric L4 L12.end A4.start
  constraint symmetric L4 L13.end A4.end
  constraint symmetric L4 A2 A4
  constraint symmetric L4 L21.start L25.start
  constraint symmetric L4 L22.start L24.start
  constraint symmetric L7 L12.end A6.start
  constraint symmetric L7 L13.end A6.end
  constraint symmetric L7 A2 A6
  constraint symmetric L7 L21.start L31.start
  constraint symmetric L7 L22.start L30.start
  constraint symmetric L7 A4.end L28.start
  constraint symmetric L7 A4.start A5.end
  constraint symmetric L7 A4 A5
  constraint symmetric L7 L25.start L27.start
  constraint tangent L22 A7
  constraint tangent L15 A7
  constraint coincident L14 A1.start
  constraint tangent L14 A8
  constraint tangent L21 A8
  constraint tangent L33 A9
  constraint tangent L34 A9
  constraint tangent L32 A10
  constraint tangent L31 A10
  constraint tangent L29 A11
  constraint tangent L30 A11
  constraint tangent L27 A12
  constraint tangent L28 A12
  constraint tangent L26 A13
  constraint tangent L25 A13
  constraint tangent L23 A14
  constraint tangent L24 A14
  measures "d118" diameter of A2
  measures "d119" distance of L18 L21
  measures "d120" distance of L20 L22
  measures "d121" radius of A7
  measures "d122" radius of A8
  measures "d123" radius of A9
  measures "d124" radius of A10
  measures "d125" radius of A11
  measures "d126" radius of A12
  measures "d127" radius of A13
  measures "d128" radius of A14
extrude "Extruir14" add sketch "Boceto10" along normal blind 1.6 separate body contours L0 L1 L2 L21 L31 | L0 L1 L2 L14 L15 A2 L21 L22 A4 L23 L24 L25 L26 L27 L28 A5 L29 L30 L31 A6 L32 L33 L34 A7 A8 A9 A10 A11 A12 A13 A14 makes body 11
sketch "Boceto11" plane through (0, 0, -10.35) normal (0, 0, 1) x (-1, 0, 0)
  circle A0 centre (-15.52, 41.73) radius 1.3
  circle A1 centre (-15.52, -19.28) radius 1.3
  circle A2 centre (15.57, 41.73) radius 1.3
  circle A3 centre (15.57, -19.28) radius 1.3
  arc A4 (19.97, 39.73) -> (13.57, 46.13) centre (13.57, 39.73) ccw
  line L0 (13.57, 46.13) -> (-13.52, 46.13)
  arc A5 (-13.52, 46.13) -> (-19.92, 39.73) centre (-13.52, 39.73) ccw
  line L1 (-19.92, 39.73) -> (-19.92, -17.28)
  arc A6 (-19.92, -17.28) -> (-13.52, -23.68) centre (-13.52, -17.28) ccw
  line L2 (-13.52, -23.68) -> (13.57, -23.68)
  arc A7 (13.57, -23.68) -> (19.97, -17.28) centre (13.57, -17.28) ccw
  line L3 (19.97, -17.28) -> (19.97, 39.73)
  line L4 (17.97, 16.225) -> (19.97, 16.225)
  line L5 (19.97, 16.225) -> (19.97, 6.225)
  line L6 (19.97, 6.225) -> (17.97, 6.225)
  line L7 (17.97, 6.225) -> (17.97, 16.225)
  line L8 (17.97, 16.225) -> (19.97, 6.225) construction
  line L9 (19.97, 16.225) -> (17.97, 6.225) construction
  line L10 (-17.92, 6.225) -> (-19.92, 6.225)
  line L11 (-19.92, 6.225) -> (-19.92, 16.225)
  line L12 (-19.92, 16.225) -> (-17.92, 16.225)
  line L13 (-17.92, 16.225) -> (-17.92, 6.225)
  line L14 (5.025, 44.13) -> (-4.975, 44.13)
  line L15 (-4.975, 44.13) -> (-4.975, 46.13)
  line L16 (-4.975, 46.13) -> (5.025, 46.13)
  line L17 (5.025, 46.13) -> (5.025, 44.13)
  line L18 (5.025, -21.68) -> (-4.975, -21.68)
  line L19 (-4.975, -21.68) -> (-4.975, -23.68)
  line L20 (-4.975, -23.68) -> (5.025, -23.68)
  line L21 (5.025, -23.68) -> (5.025, -21.68)
  point P0 (18.97, 11.225)
  dimension "d131" = 2
  dimension "d132" = 10
  dimension "d133" = 10
  dimension "d134" = 10
  dimension "d135" = 10
  dimension "d136" = 2
  dimension "d137" = 2
  dimension "d138" = 2
  constraint horizontal L4
  constraint perpendicular L4 L5
  constraint parallel L4 L6
  constraint parallel L5 L7
  constraint coincident L8 P0
  constraint coincident L9 P0
  constraint midpoint L3 L5
  constraint horizontal L10
  constraint vertical L11
  constraint horizontal L12
  constraint vertical L13
  constraint midpoint L1 L11
  constraint horizontal L14
  constraint vertical L15
  constraint horizontal L16
  constraint vertical L17
  constraint midpoint L0 L16
  constraint horizontal L18
  constraint vertical L19
  constraint horizontal L20
  constraint vertical L21
  constraint midpoint L2 L20
  measures "d131" distance of L5.end L6.end
  measures "d132" distance of L4.start L6.end
  measures "d133" distance of L18.start L18.end
  measures "d134" distance of L10.start L12.end
  measures "d135" distance of L14.start L14.end
  measures "d136" distance of L14.end L15.end
  measures "d137" distance of L11.end L12.end
  measures "d138" distance of L18.end L19.end
fillet "Empalme3" radius 1 4 edges at (-18.07, -6.225, -3.87) (-18.07, -16.225, -3.87) (-20.07, -6.225, -3.87) (-20.07, -16.225, -3.87) on bodies 4
fillet "Empalme4" radius 1 4 edges at (4.975, 21.78, -3.87) (4.975, 23.78, -3.87) (-5.025, 23.78, -3.87) (-5.025, 21.78, -3.87) on bodies 4
fillet "Empalme5" radius 1 4 edges at (18.02, -16.225, -3.87) (20.02, -16.225, -3.87) (18.02, -6.225, -3.87) (20.02, -6.225, -3.87) on bodies 4
fillet "Empalme6" radius 1 4 edges at (-5.025, -44.23, -3.87) (-5.025, -46.23, -3.87) (4.975, -44.23, -3.87) (4.975, -46.23, -3.87) on bodies 4
extrude "Extruir15" add sketch "Boceto11" along normal up to surface (3.88 mm away) separate body contours L3 L4 L5 L6 L7 | L0 L14 L15 L16 L17 | L2 L18 L19 L20 L21 | L1 L10 L11 L12 L13 makes body 12 at (1.6417, -44.13, -7.7633) makes body 13 at (-1.6917, 23.68, -7.7633) makes body 14 at (17.92, -9.5583, -7.7633) makes body 15 at (-19.97, -12.8917, -9.0567)
combine "Combinar6" operation add target body 10 tool bodies 12 13 14 15
fillet "Empalme7" radius 1 8 edges at (-5.025, 22.68, -10.35) (4.975, 22.68, -10.35) (18.92, -6.225, -10.35) (18.92, -16.225, -10.35) (4.975, -45.13, -10.35) (-5.025, -45.13, -10.35) (-18.97, -16.225, -10.35) (-18.97, -6.225, -10.35) on bodies 10
ref_plane "PlanoDeObra3" through (-0.0185, -11.216, -1.87) normal (0, 0, 1) x (-1, 0, 0)